Autodesk Fusion 360 part; units mm, degrees
(part 2 of 2)
equation "pcbMountHoles = 2 mm"
equation "ventDiameter = 3 mm"
equation "platformGrommetMountDiameter = 3.5 mm"
equation "hangerWireDiameter = 2 mm"
equation "topPillowHoleDistance = 22 mm"
equation "d1829 = height"
equation "d1833 = length"
equation "d1834 = toolDiameter"
equation "d1835 = boneCenterToHoleSide"
equation "d1836 = boneCenterToHoleBottom"
equation "d1837 = boneCenterToHoleSide"
equation "d1842 = toolDiameter"
equation "d1843 = boneCenterToHoleBottom"
equation "d1844 = boneCenterToHoleSide"
equation "d1845 = toolDiameter"
equation "d1846 = boneCenterToHoleSide"
equation "d1848 = toolDiameter"
equation "d1849 = boneCenterToHoleSide"
equation "d1850 = fingerWidth - 2 * kerf"
equation "d1862 = boneCenterToHoleSide"
equation "d1887 = toolDiameter"
equation "d1888 = boneCenterToHoleSide"
equation "d1889 = boneCenterToHoleBottom"
equation "d1890 = boneCenterToHoleSide"
equation "d1896 = toolDiameter"
equation "d1899 = toolDiameter"
equation "d1926 = thickness"
equation "d1948 = boneCenterToHoleBottom"
equation "d1949 = boneCenterToHoleSide"
equation "d1951 = boneCenterToHoleSide"
equation "d1953 = holeWidth"
equation "d1956 = fingerWidth - 2 * kerf"
equation "d1958 = boneCenterToHoleSide"
equation "d1959 = boneCenterToHoleBottom"
equation "d1960 = boneCenterToHoleBottom"
equation "d1961 = holeWidth"
equation "d1962 = fingerWidth - 2 * kerf"
equation "d1963 = length + toolDiameter"
equation "d1965 = thickness"
equation "d1975 = shouderHoleDepth"
equation "d1976 = fingerWidth - 2 * kerf"
equation "d1991 = depthCuts - 1"
equation "d1992 = 2 * fingerWidth"
equation "d1993 = 2 * fingerWidth"
equation "d2002 = heightCuts"
equation "d2004 = 2 * fingerWidth"
equation "d2012 = extraLineHeight"
equation "extraLineHeight = ( max(-appendix + ( sholderToothHeight - thickness ); 0.001 mm) )"
equation "appendix = fingerWidth - 2 * kerf"
equation "d2016 = 3 * thickness"
equation "d2017 = 3 * thickness"
equation "d2062 = appendix"
equation "d2063 = holeWidth"
equation "d2064 = thickness"
equation "d2068 = thickness"
equation "d2069 = appendix"
equation "d2071 = length / 2"
equation "d2072 = lengthCuts"
equation "d2074 = 2 * fingerWidth"
equation "d2076 = extraLineLength"
equation "extraLineLength = ( max(-appendix + ( shoulderToothLength ); 0.001 mm) )"
equation "d2079 = depthCuts"
equation "d2081 = 2 * fingerWidth"
equation "d2082 = lengthCuts"
equation "d2084 = 2 * fingerWidth"
equation "d2087 = extraLineLength"
equation "d2088 = depth"
equation "d2090 = depthCuts"
equation "d2092 = 2 * fingerWidth"
equation "d2095 = extraLineDepth"
equation "extraLineDepth = ( max(-appendix + ( shoulderToothDepth ); 0.001 mm) )"
equation "d2097 = extraLineDepth"
equation "d2098 = depth"
equation "d2102 = depth"
equation "d2103 = depth / 2"
equation "d2104 = thickness"
equation "d2106 = shoulderHoleLength"
equation "d2107 = toolDiameter"
equation "d2109 = holeWidth"
equation "d2110 = fingerWidth - 2 * kerf"
equation "d2111 = height / 2"
equation "d2112 = toolDiameter + length / 2"
equation "d2113 = height - toolDiameter"
equation "d2114 = length + toolDiameter"
equation "d2115 = thickness"
equation "d2116 = thickness"
equation "d2117 = holeWidth"
equation "d2118 = appendix"
equation "d2119 = appendix"
equation "d2122 = shoulderHoleHeight - thickness"
equation "d2124 = lengthCuts - 1"
equation "d2126 = 2 * fingerWidth"
equation "d2128 = lengthCuts - 1"
equation "d2130 = 2 * fingerWidth"
equation "d2133 = heightCuts - 1"
equation "d2135 = 2 * fingerWidth"
equation "d2137 = heightCuts - 1"
equation "d2139 = 2 * fingerWidth"
equation "d2140 = height"
equation "d2141 = depth"
equation "d2142 = toolDiameter + length"
equation "d2145 = sholderToothHeight"
equation "d2147 = depthCuts - 1"
equation "d2149 = 2 * fingerWidth"
equation "d2150 = heightCuts"
equation "d2152 = 2 * fingerWidth"
equation "d2154 = thickness"
named bodies: "Stock Body"
